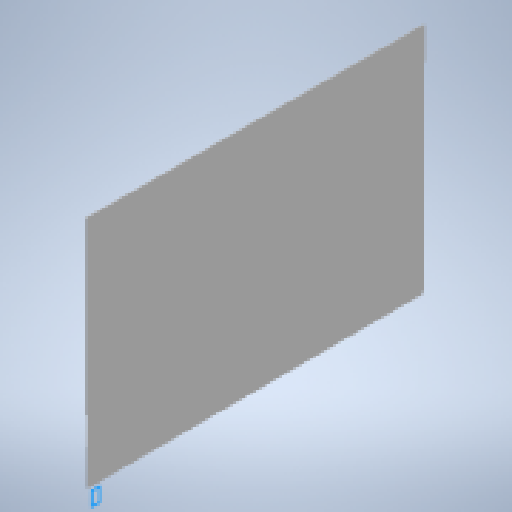
# Autodesk Inventor part: floar
Saved by Autodesk Inventor 2025.2 (Build 292293000, 293)
## iProperties
Created: 2025-06-25
Part Number: floar
Material: 一般
Document SubType Name: Modeling
Designer: naka6
Density: 1 g/cm^3
Appearance: 既定
Author: naka6
Autodesk Inventor part; units mm, degrees
ref_plane "YZ Plane" through (0, 0, 0) normal (1, 0, 0) x (0, 1, 0)
ref_plane "XZ Plane" through (0, 0, 0) normal (0, 1, 0) x (-1, 0, 0)
ref_plane "XY Plane" through (0, 0, 0) normal (0, 0, 1) x (1, 0, 0)
sketch "スケッチ1" plane through (0, 0, 0) normal (1, 0, 0) x (0, 1, 0)
  line L0 (0, 0) -> (2847.2316, 0)
  line L1 (2847.2316, 0) -> (2847.2316, -4099.8518)
  line L2 (2847.2316, -4099.8518) -> (0, -4099.8518)
  line L3 (0, -4099.8518) -> (0, 0)
  constraints: 8 end point, 2 parallel, 1 horizontal, 1 perpendicular
extrude "押し出し1" add sketch "スケッチ1" along normal blind 10
sketch "スケッチ4" plane through (0, 0, 0) normal (-1, 0, 0) x (0, 0, 1)
  line L0 (-2312.9612, 1659.4013) -> (-2006.8226, 1659.4013) construction
  line L1 (-2006.8226, 1659.4013) -> (-2006.8226, 1225.8968) construction
  line L2 (-2006.8226, 1225.8968) -> (-2312.9612, 1225.8968) construction
  line L3 (-2312.9612, 1225.8968) -> (-2312.9612, 1659.4013) construction
  point P0 (0, 0)
  constraints: 2 other
decal "デカール2"
